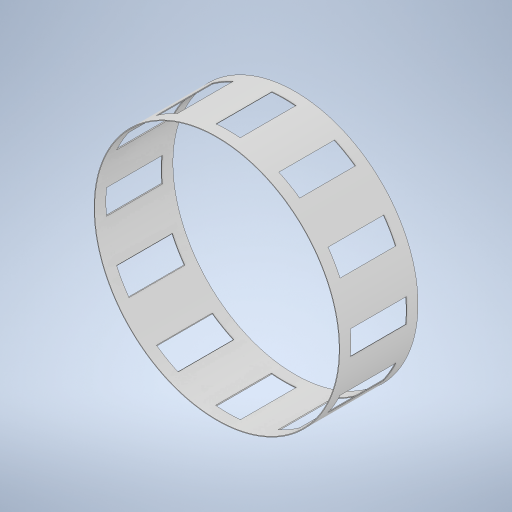
# Autodesk Inventor part: Lock
Saved by Autodesk Inventor 2023 (Build 270158000, 158)
## iProperties
Created: 2023-10-09
Part Number: Lock
Material: Generic
Document SubType Name: Modeling
Designer: huy20
Density: 1 g/cm^3
Appearance: Default
Author: huy20
Autodesk Inventor part; units mm, degrees
ref_plane "YZ Plane" through (0, 0, 0) normal (1, 0, 0) x (0, 1, 0)
ref_plane "XZ Plane" through (0, 0, 0) normal (0, 1, 0) x (-1, 0, 0)
ref_plane "XY Plane" through (0, 0, 0) normal (0, 0, 1) x (1, 0, 0)
sketch "Sketch1" plane through (0, 0, 0) normal (0, 0, 1) x (1, 0, 0)
  circle A0 centre (0, 0) radius 4.375
  circle A1 centre (0, 0) radius 4.4
  dimension "d1" = 8.75
  dimension "d2" = 8.8
  constraints: 2 centre point, 1 coincident
  measures "d1" diameter of A0
  measures "d2" diameter of A1
extrude "Extrusion1" add sketch "Sketch1" along normal mid plane 2.8
ref_plane "Work Plane1" through (0, 0, 0) normal (0, 0, 1) x (1, 0, 0)
sketch "Sketch2" plane through (0, 0, 0) normal (0, 0, 1) x (1, 0, 0)
  circle A0 centre (0, 4.125) radius 0.5
  circle A1 centre (-2.0625, 3.5724) radius 0.5
  circle A2 centre (-3.5724, 2.0625) radius 0.5
  circle A3 centre (-4.125, 0) radius 0.5
  circle A4 centre (-3.5724, -2.0625) radius 0.5
  circle A5 centre (-2.0625, -3.5724) radius 0.5
  circle A6 centre (0, -4.125) radius 0.5
  circle A7 centre (2.0625, -3.5724) radius 0.5
  circle A8 centre (3.5724, -2.0625) radius 0.5
  circle A9 centre (4.125, 0) radius 0.5
  circle A10 centre (3.5724, 2.0625) radius 0.5
  circle A11 centre (2.0625, 3.5724) radius 0.5
  point P0 (0, 0)
  dimension "d5" = 1
  dimension "d6" = 4.125
  dimension "d9" = 360
  constraints: 12 centre point, 25 other
  measures "d5" diameter of A0
  measures "d6" distance of point (0, 0) A0.centre
extrude "Extrusion2" cut sketch "Sketch2" along normal mid plane 2
body "Solid1"
